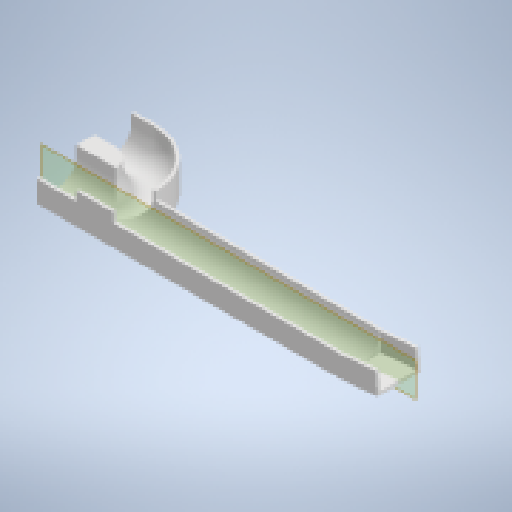
# Autodesk Inventor part: Libera todas
Saved by Autodesk Inventor 2024 (Build 280153000, 153)
## iProperties
Created: 2023-05-16
Part Number: Libera todas
Material: Genérico
Document SubType Name: Modeling
Designer: jpjoa
Density: 1 g/cm^3
Appearance: Padrão
Author: jpjoa
Autodesk Inventor part; units mm, degrees
ref_plane "YZ Plane" through (0, 0, 0) normal (1, 0, 0) x (0, 1, 0)
ref_plane "XZ Plane" through (0, 0, 0) normal (0, 1, 0) x (-1, 0, 0)
ref_plane "XY Plane" through (0, 0, 0) normal (0, 0, 1) x (1, 0, 0)
sketch "Esboço1" plane through (0, 0, 0) normal (0, 1, 0) x (-1, 0, 0)
  arc A0 (-19.6, -19.6) -> (-10.6, -28.6) centre (-10.6, -19.6) ccw
  arc A1 (-37.6, -19.6) -> (-10.6, -46.6) centre (-10.6, -19.6) ccw
  line L0 (-10.6, -46.6) -> (-1.6, -46.6)
  line L1 (-1.6, -46.6) -> (-1.6, -28.6)
  line L2 (-1.6, -28.6) -> (-10.6, -28.6)
  line L3 (-19.6, -19.6) -> (-1.6, -19.6)
  line L4 (-1.6, -19.6) -> (-1.6, -1.6)
  line L5 (-1.6, -1.6) -> (-148.4, -1.6)
  line L6 (-148.4, -1.6) -> (-148.4, -19.6)
  line L7 (-148.4, -19.6) -> (-37.6, -19.6)
  arc A2 (-39.2, -19.6) -> (-10.6, -48.2) centre (-10.6, -19.6) ccw
  line L8 (-150, -21.2) -> (-150, 0)
  line L9 (-150, 0) -> (0, 0)
  line L10 (0, 0) -> (0, -19.6)
  line L11 (0, -19.6) -> (-10.6, -19.6)
  line L12 (0, -19.6) -> (0, -48.2)
  line L13 (0, -48.2) -> (-10.6, -48.2)
  line L14 (-1.6, -28.6) -> (0, -28.6)
  line L15 (0, -46.6) -> (-1.6, -46.6)
  line L16 (0, -19.6) -> (-1.6, -19.6)
  line L17 (0, -1.6) -> (-1.6, -1.6)
  line L18 (-148.4, -19.6) -> (-150, -19.6)
  line L19 (-148.4, -1.6) -> (-150, -1.6)
  line L20 (-10.6, -48.2) -> (-10.6, -46.6)
  line L21 (-150, -21.2) -> (-39.1552, -21.2)
  line L22 (-19.6, -1.6) -> (-19.6, 0)
  line L23 (-37.6, -1.6) -> (-37.6, 0)
  point P0 (-1.6, -19.6)
  point P1 (-10.6, -48.2)
  dimension "d7" = 18
  dimension "d8" = 9
  dimension "d9" = 18
  dimension "d11" = 9
  dimension "d12" = 1.6
  dimension "d13" = 150
  dimension "d14" = 1.6
  dimension "d15" = 1.6
  constraints: 48 end point, 17 point on line, 10 coincident, 9 horizontal, 9 point on circle, 7 perpendicular, 5 vertical alignment, 4 vertical, 3 centre point, 3 horizontal alignment, 3 other
  measures "d7" radial gap between concentric circles of A0 A1
  measures "d8" distance of L0.start L0.end
  measures "d9" distance of L5.end L6.end
  measures "d11" distance between parallel lines of L3 L2
  measures "d12" radial gap between concentric circles of A1 A2
  measures "d13" distance of L8.end L9.end
  measures "d14" distance between parallel lines of L12 L1
  measures "d15" distance between parallel lines of L7 L21
extrude "Extrusão1" add sketch "Esboço1" against normal blind 1.6
extrude "Extrusão2" add sketch "Esboço1" along normal blind 9 contours L5 L22 L9 L10 L17 | L5 L19 L8 L9 L23 | A2 L21 L8 L18 L7
extrude "Extrusão3" add sketch "Esboço1" along normal blind 13.5 contours L3 L11 L12 L14 L2 A0 | L15 L12 L13 L20 L0 | L20 A2 L7 A1 | L5 L23 L9 L22
fillet "Arredondamento1" radius 9 7 edges at (5.3, 0, -46.6) (29.6919, 0, -38.6919) (16.964, 0, -25.964) (5.3, 0, -28.6) (9.8, 0, -19.6) (93.8, 0, -19.6) (75, 0, -1.6)
sketch "Esboço2" plane through (0, -1.6, 0) normal (0, 0, 1) x (1, 0, 0)
  line L0 (150, 0) -> (0, 0) projected
  line L1 (150, 0) -> (159.9619, 0.8716)
  line L2 (150, 0) -> (160, 0) construction
  line L3 (159.9619, 0.8716) -> (159.0416, 11.391)
  line L4 (37.6, 10.6) -> (150, 10.6) projected
  line L5 (159.0416, 11.391) -> (150, 10.6)
  line L6 (150, 1.6) -> (150, 10.6) projected
  line L7 (150, 0) -> (150, 10.6)
  point P0 (0, 1.6)
  dimension "d23" = 10
  dimension "d24" = 5
  dimension "d25" = 5
  constraints: 10 end point, 1 collinear, 1 equal length, 1 horizontal, 1 perpendicular
  measures "d23" distance of L0.start L1.end
  measures "d24" angle of L2 L1
  measures "d25" angle of L4 L5
extrude "Extrusão4" add sketch "Esboço2" against normal up to surface (21.2 mm away)
ref_plane "Plano de trabalho1" through (39.1552, -1.6, -10.6) normal (0, 0, -1) x (-1, 0, 0)
sketch "Esboço3" plane through (39.1552, -1.6, -10.6) normal (0, 0, -1) x (-1, 0, 0)
  line L0 (1.5552, 10.6) -> (-110.8448, 10.6) projected
  line L1 (-119.8864, 11.391) -> (-110.8448, 10.6) projected
  line L2 (-120.6708, 2.4253) -> (-111.2377, 1.6)
  line L3 (-111.2377, 1.6) -> (1.5552, 1.6)
  line L4 (-120.8067, 0.8716) -> (-119.8864, 11.391) projected
  line L5 (-120.6708, 2.4253) -> (-119.8864, 11.391)
  line L6 (-119.8864, 11.391) -> (-110.8448, 10.6)
  line L7 (-110.8448, 1.5656) -> (-110.8448, 10.6)
  line L8 (39.1552, 1.6) -> (-110.8448, 1.6) projected
  point P0 (39.1552, 1.6)
  point P1 (-110.8448, 1.6)
  dimension "d28" = 9
  constraints: 10 end point, 2 collinear, 1 perpendicular, 1 other
  measures "d28" distance between parallel lines of L1 L2
extrude "Extrusão5" cut sketch "Esboço3" along normal mid plane 18
fillet "Arredondamento2" radius 9 2 edges at (155.1095, 0.4126, -19.6) (155.1095, 0.4126, -1.6)
equation "\"d7\" = Esfera"
equation "\"d8\" = 0.5 * Esfera"
equation "\"d9\" = Esfera"
equation "\"d12\" = Margem"
equation "\"d14\" = Margem"
equation "\"d15\" = Margem"
equation "\"d16\" = Margem"
equation "\"d18\" = 0.5 * Esfera"
equation "\"d20\" = 0.75 * Esfera"
equation "\"d22\" = 0.5 * Esfera"
equation "\"d28\" = 0.5 * Esfera"
equation "\"d29\" = Esfera"
equation "\"d31\" = 0.5 * Esfera"
equation "\"Esfera\" = 18"
equation "\"Margem\" = 1.6"
